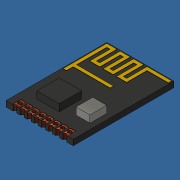
# Autodesk Inventor part: nRF24L01+_SMD
Saved by Autodesk Inventor 2018 (Build 220112000, 112)
## iProperties
Created: 2017-12-09
Part Number: nRF24L01+_SMD
Material: Generisch
Document SubType Name: Modeling
Designer: Martin
Density: 1 g/cm^3
Appearance: Gummi - schwarz
Author: Martin
Autodesk Inventor part; units mm, degrees
ref_plane "YZ Plane" through (0, 0, 0) normal (1, 0, 0) x (0, 1, 0)
ref_plane "XZ Plane" through (0, 0, 0) normal (0, 1, 0) x (-1, 0, 0)
ref_plane "XY Plane" through (0, 0, 0) normal (0, 0, 1) x (1, 0, 0)
sketch "Skizze1" plane through (0, 0, 0) normal (0, 0, 1) x (1, 0, 0)
  line L0 (-6, 18) -> (6, 18)
  line L1 (6, 18) -> (6, 0)
  line L2 (6, 0) -> (-6, 0)
  line L3 (-6, 0) -> (-6, 18)
  point P0 (0, 0)
  point P1 (0, 0)
  dimension "d0" = 12
  dimension "d1" = 18
  constraints: 8 end point, 2 parallel, 1 coincident, 1 horizontal, 1 midpoint, 1 perpendicular
  measures "d0" distance of L1.end L2.end
  measures "d1" distance of L0.end L1.end
extrude "Extrusion1" add sketch "Skizze1" along normal blind 1
sketch "Skizze2" plane through (0, 0, 1) normal (0, 0, 1) x (1, 0, 0)
  line L0 (-4.85, 0) -> (-3.95, 0)
  line L1 (-3.95, 0) -> (-3.95, 1.5)
  line L2 (-3.95, 1.5) -> (-4.85, 1.5)
  line L3 (-4.85, 1.5) -> (-4.85, 0)
  line L4 (-4.4, 1.5) -> (-4.4, 0) construction
  line L5 (-6, 18) -> (-6, 0) construction
  circle A0 centre (-4.4, 0.9) radius 0.35 construction
  circle A1 centre (-4.4, 0) radius 0.35 construction
  point P0 (0, 0)
  dimension "d4" = 1.6
  dimension "d5" = 0.9
  dimension "d6" = 0.7
  dimension "d7" = 0.9
  dimension "d8" = 1.5
  constraints: 10 end point, 2 centre point, 2 midpoint, 2 parallel, 2 point on line, 1 coincident, 1 equal radius, 1 horizontal, 1 perpendicular
  measures "d4" distance between parallel lines of L5 L4
  measures "d5" distance of L1.end L2.end
  measures "d6" diameter of A0
  measures "d7" distance from line of L0 A0.centre
  measures "d8" distance of L0.end L1.end
extrude "Extrusion2" cut sketch "Skizze2" against normal blind 0.05
hole "Bohrung1" at (-4.4, 0.9, 1) at (-4.4, 0, 1) direction (0, 0, -1) diameter 0.7 end through all
pattern_linear "Rechteckige Anordnung1" count 8 spacing 1.27 along (1, 0, 0) of "Extrusion2", "Bohrung1"
sketch "Skizze3" plane through (0, 0, 1) normal (0, 0, 1) x (1, 0, 0)
  line L0 (-5.8, 10) -> (-5.8, 17.8)
  line L1 (-5.8, 17.8) -> (-4, 17.8)
  line L2 (-4, 17.8) -> (-4, 14.15)
  line L3 (-4, 14.15) -> (-3.4, 14.15)
  line L4 (-3.4, 14.15) -> (-3.4, 17.8)
  line L5 (-3.4, 17.8) -> (-1.6, 17.8)
  line L6 (-1.6, 17.8) -> (-1.6, 14.15)
  line L7 (-1.6, 14.15) -> (-1, 14.15)
  line L8 (-1, 14.15) -> (-1, 17.8)
  line L9 (-1, 17.8) -> (0.8, 17.8)
  line L10 (0.8, 17.8) -> (0.8, 14.15)
  line L11 (0.8, 14.15) -> (1.4, 14.15)
  line L12 (1.4, 14.15) -> (1.4, 17.8)
  line L13 (1.4, 17.8) -> (5.8, 17.8)
  line L14 (5.8, 17.8) -> (5.8, 17.2)
  line L15 (5.8, 17.2) -> (2, 17.2)
  line L16 (2, 17.2) -> (2, 13.55)
  line L17 (2, 13.55) -> (0.2, 13.55)
  line L18 (0.2, 13.55) -> (0.2, 17.2)
  line L19 (0.2, 17.2) -> (-0.4, 17.2)
  line L20 (-0.4, 17.2) -> (-0.4, 13.55)
  line L21 (-0.4, 13.55) -> (-2.2, 13.55)
  line L22 (-2.2, 13.55) -> (-2.2, 17.2)
  line L23 (-2.2, 17.2) -> (-2.8, 17.2)
  line L24 (-2.8, 17.2) -> (-2.8, 13.55)
  line L25 (-2.8, 13.55) -> (-4.6, 13.55)
  line L26 (-4.6, 13.55) -> (-4.6, 17.2)
  line L27 (-4.6, 17.2) -> (-5.2, 17.2)
  line L28 (-5.2, 17.2) -> (-5.2, 11.8)
  line L29 (-5.2, 11.8) -> (1.4, 11.8)
  line L30 (1.4, 11.8) -> (1.4, 11.2)
  line L31 (1.4, 11.2) -> (-5.2, 11.2)
  line L32 (-5.2, 11.2) -> (-5.2, 10)
  line L33 (-5.2, 10) -> (-5.8, 10)
  line L34 (-6, 18) -> (-6, 0) projected
  line L35 (6, 0) -> (6, 18) projected
  point P0 (0, 0)
  point P1 (1.4, 11.5)
  dimension "d21" = 0.2
  dimension "d22" = 0.2
  dimension "d23" = 0.2
  dimension "d24" = 11.5
  dimension "d25" = 0.6
  dimension "d26" = 0.6
  dimension "d27" = 0.6
  dimension "d28" = 0.6
  dimension "d29" = 0.6
  dimension "d30" = 0.6
  dimension "d31" = 4.25
  dimension "d32" = 0
  dimension "d33" = 10
  constraints: 68 end point, 23 perpendicular, 18 point on line, 10 equal length, 2 collinear, 1 midpoint, 1 parallel, 1 vertical
  measures "d21" distance between parallel lines of L34 L0
  measures "d22" distance between parallel lines of L35 L14
  measures "d23" distance from line of L34.start L1
  measures "d24" vertical distance of point (0, 0) point (1.4, 11.5)
  measures "d25" distance of L32.end L0.start
  measures "d26" distance between parallel lines of L26 L2
  measures "d27" distance between parallel lines of L24 L4
  measures "d28" distance between parallel lines of L25 L3
  measures "d29" distance between parallel lines of L6 L22
  measures "d30" distance between parallel lines of L10 L18
  measures "d31" distance between parallel lines of L13 L17
  measures "d32" distance between parallel lines of L12 L30
  measures "d33" distance from line of point (0, 0) L33
extrude "Extrusion3" add sketch "Skizze3" along normal blind 0.05
sketch "Skizze4" plane through (0, 0, 1) normal (0, 0, 1) x (1, 0, 0)
  line L0 (-3.5, 7) -> (0.5, 7)
  line L1 (0.5, 7) -> (0.5, 3)
  line L2 (0.5, 3) -> (-3.5, 3)
  line L3 (-3.5, 3) -> (-3.5, 7)
  line L4 (-6, 18) -> (-6, 0) projected
  point P0 (0, 0)
  dimension "d36" = 3
  dimension "d37" = 2.5
  dimension "d38" = 4
  dimension "d39" = 4
  constraints: 8 end point, 2 parallel, 1 horizontal, 1 perpendicular
  measures "d36" distance from line of point (0, 0) L2
  measures "d37" distance between parallel lines of L4 L3
  measures "d38" distance of L0.start L0.end
  measures "d39" distance of L2.end L0.start
extrude "Extrusion4" add sketch "Skizze4" along normal blind 1.27
sketch "Skizze5" plane through (0, 0, 1) normal (0, 0, 1) x (1, 0, 0)
  line L0 (5, 7) -> (2.5, 7)
  line L1 (2.5, 7) -> (2.5, 4)
  line L2 (2.5, 4) -> (5, 4)
  line L3 (5, 4) -> (5, 7)
  line L4 (6, 0) -> (6, 18) projected
  point P0 (0, 0)
  dimension "d42" = 3
  dimension "d43" = 2.5
  dimension "d44" = 4
  dimension "d45" = 1
  constraints: 8 end point, 2 parallel, 1 horizontal, 1 perpendicular
  measures "d42" distance of L2.end L0.start
  measures "d43" distance of L0.start L0.end
  measures "d44" distance from line of point (0, 0) L2
  measures "d45" distance between parallel lines of L4 L3
extrude "Extrusion5" add sketch "Skizze5" along normal blind 1.27
equation "\"d11\" = d6"
equation "\"d22\" = d21"
equation "\"d23\" = d21"
equation "\"d26\" = d25"
equation "\"d27\" = d25"
equation "\"d28\" = d25"
equation "\"d29\" = d27"
equation "\"d30\" = d29"
